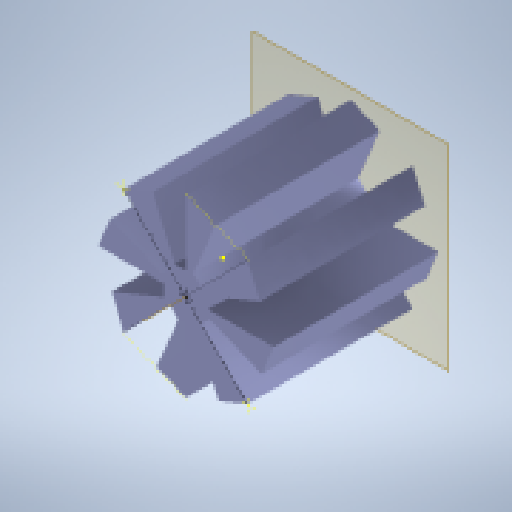
# Autodesk Inventor part: dopychacz
Saved by Autodesk Inventor 2023 (Build 270158000, 158)
## iProperties
Created: 2022-05-03
Part Number: dopychacz
Material: Ogólny
Document SubType Name: Modeling
Designer: Ciućmok
Density: 1 g/cm^3
Appearance: Chrom — niebieski polerowany
Author: Ciućmok
Autodesk Inventor part; units mm, degrees
ref_plane "YZ Plane" through (0, 0, 0) normal (1, 0, 0) x (0, 1, 0)
ref_plane "XZ Plane" through (0, 0, 0) normal (0, 1, 0) x (-1, 0, 0)
ref_plane "XY Plane" through (0, 0, 0) normal (0, 0, 1) x (1, 0, 0)
ref_plane "Płaszczyzna konstrukcyjna1" through (0, 0, 0) normal (0, 0, 1) x (1, 0, 0)
sketch "Szkic1" plane through (0, 0, 0) normal (0, 0, 1) x (1, 0, 0)
  line L0 (8.0251, 3.4329) -> (-11.0866, 11.3492) projected
  line L1 (-11.0866, 11.3492) -> (-30.1982, 3.4329) projected
  line L2 (-30.1982, 3.4329) -> (-38.1145, -15.6788) projected
  line L3 (-38.1145, -15.6788) -> (-30.1982, -34.7904) projected
  line L4 (-30.1982, -34.7904) -> (-11.0866, -42.7067) projected
  line L5 (-11.0866, -42.7067) -> (8.0251, -34.7904) projected
  line L6 (8.0251, -34.7904) -> (15.9414, -15.6788) projected
  line L7 (15.9414, -15.6788) -> (8.0251, 3.4329) projected
  point P0 (0, 0)
extrude "Wyciągnięcie proste1" add sketch "Szkic1" along normal blind 50
sketch "Szkic2" plane through (0, 0, 50) normal (0, 0, 1) x (1, 0, 0)
  line L0 (-35.3977, -2.8484) -> (-36.8759, -2.2361) projected
  line L1 (-31.4727, 0.356) -> (-35.1682, 1.8867) projected
  line L2 (8.0251, 3.4329) -> (-11.0866, 11.3492) construction
  line L3 (8.0251, 3.4329) -> (-30.1982, -34.7904) construction
  line L4 (-11.0866, 11.3492) -> (-30.1982, 3.4329) construction
  line L5 (-11.0866, -42.7067) -> (8.0251, -34.7904) construction
  line L6 (-30.1982, 3.4329) -> (8.0251, -34.7904) construction
  line L7 (-30.1982, 3.4329) -> (-38.1145, -15.6788) projected
  line L8 (-30.1982, 3.4329) -> (-15.8633, -10.902)
  line L9 (-15.8633, -10.902) -> (-18.3147, -13.3534)
  line L10 (-18.3147, -13.3534) -> (-34.3927, -6.6936)
  line L11 (-30.1982, 3.4329) -> (-34.3927, -6.6936)
  line L12 (-38.1145, -15.6788) -> (-30.1982, -34.7904) projected
  line L13 (-34.0232, -6.8467) -> (-37.6815, -15.6788)
  line L14 (-38.1145, -15.6788) -> (-11.0866, -15.6788)
  point P0 (0, 0)
  dimension "d7" = 0.4
  constraints: 16 end point, 4 point on line, 3 perpendicular, 1 midpoint, 1 parallel
  measures "d7" distance between parallel lines of L7 L13
extrude "Wyciągnięcie proste2" cut sketch "Szkic2" against normal through all
sketch "Szkic3" plane through (0, 0, 50) normal (0, 0, 1) x (1, 0, 0)
  line L0 (8.0251, 3.4329) -> (-11.0866, 11.3492) construction
  line L1 (-30.1982, -34.7904) -> (-11.0866, -42.7067) construction
  line L2 (8.0251, 3.4329) -> (-30.1982, -34.7904) construction
  line L3 (8.0251, -34.7904) -> (-30.1982, 3.4329) construction
  point P0 (0, 0)
  point P1 (-11.0866, -15.6788)
  constraints: 4 end point, 2 coincident, 2 midpoint
pattern_circular "Szyk kołowy1" count 8 over 360 about axis through (-11.0866, -15.6788, 50) along (0, 0, 1) of "Wyciągnięcie proste2"
